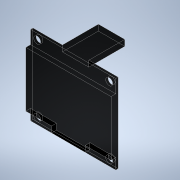
# Autodesk Inventor part: display
Saved by Autodesk Inventor 2021 (Build 250183000, 183)
## iProperties
Created: 2021-12-17
Part Number: display
Material: Glas
Document SubType Name: Modeling
Designer: Tilman Preuschoff
Density: 0.1 g/cm^3
Appearance: Klar
Author: Tilman Preuschoff
Autodesk Inventor part; units mm, degrees
ref_plane "YZ Plane" through (0, 0, 0) normal (1, 0, 0) x (0, 1, 0)
ref_plane "XZ Plane" through (0, 0, 0) normal (0, 1, 0) x (-1, 0, 0)
ref_plane "XY Plane" through (0, 0, 0) normal (0, 0, 1) x (1, 0, 0)
sketch "Skizze1" plane through (0, 0, 0) normal (0, 0, 1) x (1, 0, 0)
  line L0 (-17.75, 16.5) -> (17.75, 16.5)
  line L1 (17.75, 16.5) -> (17.75, -16.5)
  line L2 (17.75, -16.5) -> (-17.75, -16.5)
  line L3 (-17.75, -16.5) -> (-17.75, 16.5)
  line L4 (-17.75, 16.5) -> (17.75, -16.5) construction
  line L5 (17.75, 16.5) -> (-17.75, -16.5) construction
  point P0 (0, 0)
  dimension "d0" = 33
  dimension "d1" = 35.5
  constraints: 12 end point, 2 midpoint, 2 parallel, 1 horizontal, 1 perpendicular
  measures "d0" distance between parallel lines of L2 L0
  measures "d1" distance between parallel lines of L1 L3
extrude "Extrusion1" add sketch "Skizze1" along normal blind 1
sketch "Skizze2" plane through (0, 0, 1) normal (0, 0, 1) x (1, 0, 0)
  line L0 (-17.75, 16.5) -> (-17.75, -16.5) projected
  line L1 (17.75, -16.5) -> (17.75, 16.5) projected
  line L2 (-17.75, 11) -> (17.75, 11)
  line L3 (17.75, 11) -> (17.75, -12)
  line L4 (17.75, -12) -> (-17.75, -12)
  line L5 (-17.75, -12) -> (-17.75, 11)
  line L6 (17.75, 16.5) -> (-17.75, 16.5) projected
  line L7 (-7, -14.5) -> (7, -14.5)
  line L8 (7, -14.5) -> (7, -12)
  line L9 (7, -12) -> (-7, -12)
  line L10 (-7, -12) -> (-7, -14.5)
  line L11 (-7, -14.5) -> (7, -12) construction
  line L12 (7, -14.5) -> (-7, -12) construction
  line L13 (-17.75, -16.5) -> (17.75, -16.5) projected
  point P0 (0, 0)
  point P1 (0, -13.25)
  point P2 (0, -13.25)
  point P3 (17.75, 11)
  point P4 (-17.75, -12)
  point P5 (-7, -12)
  dimension "d4" = 23
  dimension "d5" = 5.5
  dimension "d6" = 14
  dimension "d7" = 2
  constraints: 20 end point, 4 parallel, 3 midpoint, 3 point on line, 2 horizontal, 2 perpendicular, 1 vertical alignment
  measures "d4" distance between parallel lines of L4 L2
  measures "d5" distance between parallel lines of L2 L6
  measures "d6" distance between parallel lines of L8 L10
  measures "d7" distance between parallel lines of L13 L7
extrude "Extrusion2" add sketch "Skizze2" along normal blind 2 contours L2 L1 L4 L0 | L4 L8 L7 L10
sketch "Skizze3" plane through (0, 0, 0) normal (0, 0, -1) x (-1, 0, 0)
  line L0 (-17.75, 16.5) -> (17.75, 16.5) projected
  line L1 (-5.5, 14) -> (5.5, 14)
  line L2 (5.5, 14) -> (5.5, 16.5)
  line L3 (5.5, 16.5) -> (-5.5, 16.5)
  line L4 (-5.5, 16.5) -> (-5.5, 14)
  line L5 (-5.5, 14) -> (5.5, 16.5) construction
  line L6 (5.5, 14) -> (-5.5, 16.5) construction
  point P0 (0, 0)
  point P1 (0, 15.25)
  point P2 (0, 15.25)
  dimension "d10" = 11
  dimension "d11" = 2.5
  constraints: 12 end point, 3 midpoint, 2 parallel, 1 horizontal, 1 perpendicular, 1 point on line, 1 vertical alignment
  measures "d10" distance between parallel lines of L2 L4
  measures "d11" distance between parallel lines of L0 L1
extrude "Extrusion3" add sketch "Skizze3" along normal blind 15
sketch "Skizze4" plane through (0, 0, 1) normal (0, 0, 1) x (1, 0, 0)
  line L0 (-15, 14) -> (15, 14)
  line L1 (15, 14) -> (15, -14)
  line L2 (15, -14) -> (-15, -14)
  line L3 (-15, -14) -> (-15, 14)
  line L4 (-15, 14) -> (15, -14) construction
  line L5 (15, 14) -> (-15, -14) construction
  point P0 (0, 0)
  dimension "d14" = 28
  dimension "d15" = 30
  constraints: 12 end point, 2 midpoint, 2 parallel, 1 horizontal, 1 perpendicular
  measures "d14" distance between parallel lines of L2 L0
  measures "d15" distance between parallel lines of L1 L3
hole "Bohrung1" at (-15, 14, 1) at (15, 14, 1) at (15, -14, 1) at (-15, -14, 1) direction (0, 0, -1) diameter 2.9 end through all clearance for "Flachkopfsenkschraube ISO 2009/7046" size "M2.5" standard "ISO"
